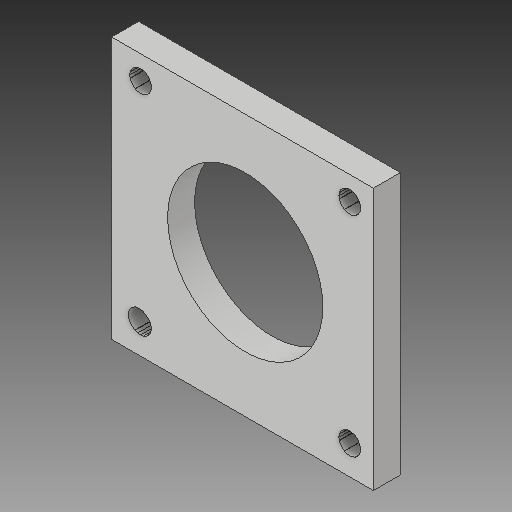
# Autodesk Inventor part: F608Brace
Saved by Autodesk Inventor 2018 (Build 220112000, 112)
## iProperties
Created: 2018-05-15
Part Number: F608Brace
Material: Generic
Document SubType Name: Modeling
Designer: Dan
Density: 1 g/cm^3
Appearance: Default
Author: Dan
Autodesk Inventor part; units mm, degrees
ref_plane "YZ Plane" through (0, 0, 0) normal (1, 0, 0) x (0, 1, 0)
ref_plane "XZ Plane" through (0, 0, 0) normal (0, 1, 0) x (-1, 0, 0)
ref_plane "XY Plane" through (0, 0, 0) normal (0, 0, 1) x (1, 0, 0)
sketch "Sketch1" plane through (0, 0, 0) normal (0, 0, 1) x (1, 0, 0)
  arc A0 (13.943993, 13.350074) -> (15.524314, 13.350965) centre (14.733369, 14.741794) ccw
  line L0 (13.943993, 13.350074) -> (13.933331, 13.354339)
  line L1 (13.933331, 13.354339) -> (13.923526, 13.361883)
  arc A1 (13.193242, 14.308193) -> (13.923526, 13.361883) centre (14.733369, 14.741794) ccw
  line L2 (13.193242, 14.308193) -> (13.18334, 14.329416)
  line L3 (13.18334, 14.329416) -> (13.179439, 14.360609)
  arc A2 (13.133423, 14.728576) -> (13.179439, 14.360609) centre (14.733369, 14.741794) ccw
  line L4 (13.133423, 14.728576) -> (13.133321, 14.729392)
  line L5 (13.133321, 14.729392) -> (13.133411, 14.730154)
  arc A3 (13.179822, 15.124538) -> (13.133411, 14.730154) centre (14.733369, 14.741794) ccw
  line L6 (13.179822, 15.124538) -> (13.18334, 15.15443)
  line L7 (13.18334, 15.15443) -> (13.193426, 15.176047)
  arc A4 (15.542796, 13.36164) -> (13.193426, 15.176047) centre (14.733369, 14.741794) ccw
  line L8 (15.542796, 13.36164) -> (15.533297, 13.354333)
  line L9 (15.533297, 13.354333) -> (15.524314, 13.350965)
  arc A5 (13.943929, -17.649894) -> (15.524326, -17.649018) centre (14.733356, -16.258203) ccw
  line L10 (13.943929, -17.649894) -> (13.933313, -17.645647)
  line L11 (13.933313, -17.645647) -> (13.923549, -17.638135)
  arc A6 (13.193209, -16.691733) -> (13.923549, -17.638135) centre (14.733356, -16.258203) ccw
  line L12 (13.193209, -16.691733) -> (13.183342, -16.670586)
  line L13 (13.183342, -16.670586) -> (13.179457, -16.639513)
  arc A7 (13.133409, -16.271293) -> (13.179457, -16.639513) centre (14.733356, -16.258203) ccw
  line L14 (13.133409, -16.271293) -> (13.133319, -16.270568)
  line L15 (13.133319, -16.270568) -> (13.133398, -16.26989)
  arc A8 (13.179821, -15.875412) -> (13.133398, -16.26989) centre (14.733356, -16.258203) ccw
  line L16 (13.179821, -15.875412) -> (13.183332, -15.845572)
  line L17 (13.183332, -15.845572) -> (13.193401, -15.823993)
  arc A9 (15.542786, -17.638356) -> (13.193401, -15.823993) centre (14.733356, -16.258203) ccw
  line L18 (15.542786, -17.638356) -> (15.533298, -17.645654)
  line L19 (15.533298, -17.645654) -> (15.524326, -17.649018)
  arc A10 (-17.056055, 13.35011) -> (-15.475745, 13.350946) centre (-16.266635, 14.741806) ccw
  line L20 (-17.056055, 13.35011) -> (-17.066673, 13.354358)
  line L21 (-17.066673, 13.354358) -> (-17.07644, 13.361872)
  arc A11 (-17.806789, 14.3083) -> (-17.07644, 13.361872) centre (-16.266635, 14.741806) ccw
  line L22 (-17.806789, 14.3083) -> (-17.816641, 14.329416)
  line L23 (-17.816641, 14.329416) -> (-17.820521, 14.360441)
  arc A12 (-17.866582, 14.728771) -> (-17.820521, 14.360441) centre (-16.266635, 14.741806) ccw
  line L24 (-17.866582, 14.728771) -> (-17.86666, 14.729392)
  line L25 (-17.86666, 14.729392) -> (-17.866592, 14.729972)
  arc A13 (-17.820136, 15.124738) -> (-17.866592, 14.729972) centre (-16.266635, 14.741806) ccw
  line L26 (-17.820136, 15.124738) -> (-17.816641, 15.15443)
  line L27 (-17.816641, 15.15443) -> (-17.806622, 15.175905)
  arc A14 (-15.457117, 13.361704) -> (-17.806622, 15.175905) centre (-16.266635, 14.741806) ccw
  line L28 (-15.457117, 13.361704) -> (-15.466692, 13.35434)
  line L29 (-15.466692, 13.35434) -> (-15.475745, 13.350946)
  circle A15 centre (-13.085739, 32.480726) radius 6.1
  circle A16 centre (48.058188, -36.595465) radius 2.65
  circle A17 centre (-36.59155, 13.204403) radius 2.65
  circle A18 centre (-36.591601, 48.078292) radius 2.65
  circle A19 centre (13.208377, -36.595598) radius 2.65
  circle A20 centre (32.483633, -13.170492) radius 6.1
  circle A21 centre (-0.766671, -0.770593) radius 16.1
  arc A22 (-15.450777, -14.918736) -> (-17.090909, -17.618262) centre (-16.489787, -16.135477) ccw
  line L30 (-15.450777, -14.918736) -> (-15.134734, -15.144406)
  line L31 (-15.134734, -15.144406) -> (-14.884762, -15.469407)
  line L32 (-14.884762, -15.469407) -> (-14.734795, -15.844416)
  line L33 (-14.734795, -15.844416) -> (-14.684917, -16.269138)
  line L34 (-14.684917, -16.269138) -> (-14.734975, -16.669476)
  line L35 (-14.734975, -16.669476) -> (-14.884982, -17.044468)
  line L36 (-14.884982, -17.044468) -> (-15.13501, -17.369426)
  line L37 (-15.13501, -17.369426) -> (-15.484998, -17.644458)
  line L38 (-15.484998, -17.644458) -> (-15.860025, -17.794432)
  line L39 (-15.860025, -17.794432) -> (-16.259998, -17.84445)
  line L40 (-16.259998, -17.84445) -> (-16.685013, -17.794434)
  line L41 (-16.685013, -17.794434) -> (-17.060005, -17.644427)
  line L42 (-17.060005, -17.644427) -> (-17.090909, -17.618262)
  line L43 (-46.80313, 83.254846) -> (-48.803137, 83.254408)
  line L44 (-48.803137, 83.254408) -> (-48.780176, -21.595606)
  line L45 (-48.780176, -21.595606) -> (-21.580157, -21.58965)
  line L46 (-21.580157, -21.58965) -> (-21.5742, -48.789625)
  line L47 (-21.5742, -48.789625) -> (83.275782, -48.766664)
  line L48 (83.275782, -48.766664) -> (83.275344, -46.766667)
  line L49 (83.275344, -46.766667) -> (-46.80313, 83.254846)
  line L50 (18.236107, 18.244089) -> (-20.563893, 18.244089)
  line L51 (-20.563893, 18.244089) -> (-20.563893, -20.572908)
  line L52 (-20.563893, -20.572908) -> (18.236107, -20.572908)
  line L53 (18.236107, -20.572908) -> (18.236107, 18.244089)
  circle A23 centre (-0.766671, -0.770593) radius 11.5
  point P0 (0, 0)
  dimension "d0" = 38.8
  dimension "d3" = 23
  constraints: 8 end point, 2 parallel, 1 centre point, 1 coincident, 1 horizontal, 1 midpoint, 1 perpendicular
  measures "d0" distance of L52.end L51.end
  measures "d3" diameter of A23
extrude "Extrusion1" add sketch "Sketch1" along normal blind 4 contours A21 | L53 L52 L51 L50
body "Solid1"
